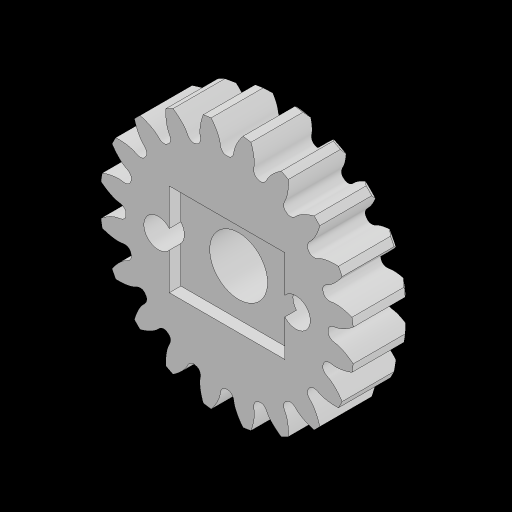
# Autodesk Inventor part: Servo Gear
Saved by Autodesk Inventor 2023.2 (Build 272271030, 271C)
## iProperties
Created: 2023-11-19
Part Number: Servo Gear
Material: Generic
Document SubType Name: Modeling
Designer: robpl
Density: 1 g/cm^3
Appearance: Default
Author: robpl
## iProperties of the stored document Servo Gear_3DPrint.ipt
Created: 2023-11-27
Part Number: Servo Gear_3DPrint
Material: Generic
Document SubType Name: Modeling
Designer: robpl
Density: 1 g/cm^3
Appearance: Default
Author: robpl
Autodesk Inventor part; units mm, degrees
ref_plane "YZ Plane" through (0, 0, 0) normal (1, 0, 0) x (0, 1, 0)
ref_plane "XZ Plane" through (0, 0, 0) normal (0, 1, 0) x (-1, 0, 0)
ref_plane "XY Plane" through (0, 0, 0) normal (0, 0, 1) x (1, 0, 0)
sketch "Sketch1" plane through (0, 0, 0) normal (0, 0, 1) x (1, 0, 0)
  spline S0 degree 3 poles (-1.3768, 10.9135) (-1.3419, 10.869) (-1.2721, 10.78) (-1.173, 10.6424) (-1.0781, 10.5017) (-0.9884, 10.3578) (-0.9041, 10.2106) (-0.826, 10.06) (-0.7548, 9.906) (-0.6919, 9.7484) (-0.6476, 9.6141) (-0.6191, 9.5046) (-0.6016, 9.4215) (-0.5932, 9.3371) (-0.5774, 9.2537) (-0.5568, 9.1714) (-0.5289, 9.0912) (-0.4924, 9.0144) (-0.4469, 8.9426) (-0.4, 8.8894) (-0.3582, 8.8513) (-0.3238, 8.8264) (-0.2881, 8.8034) (-0.2496, 8.7854) (-0.2102, 8.7696) (-0.169, 8.7594) (-0.1272, 8.7515) (-0.0706, 8.7491) (0, 8.7506) (0.0706, 8.7491) (0.1272, 8.7515) (0.169, 8.7594) (0.2102, 8.7696) (0.2496, 8.7854) (0.2881, 8.8034) (0.3238, 8.8264) (0.3582, 8.8513) (0.4, 8.8894) (0.4469, 8.9426) (0.4924, 9.0144) (0.5289, 9.0912) (0.5568, 9.1714) (0.5774, 9.2537) (0.5932, 9.3371) (0.6016, 9.4215) (0.6191, 9.5046) (0.6476, 9.6141) (0.6919, 9.7484) (0.7548, 9.906) (0.826, 10.06) (0.9041, 10.2106) (0.9884, 10.3578) (1.0781, 10.5017) (1.173, 10.6424) (1.2721, 10.78) (1.3419, 10.869) (1.3768, 10.9135) knots 0 0 0 0 0.01696 0.03392 0.050881 0.067841 0.084801 0.101761 0.11872 0.135679 0.152636 0.161116 0.169595 0.178075 0.186555 0.195032 0.203511 0.211989 0.220465 0.228938 0.233179 0.237417 0.241658 0.245897 0.250137 0.254376 0.258616 0.262855 0.271335 0.279816 0.284054 0.288295 0.292534 0.296774 0.301013 0.305254 0.309492 0.313732 0.322205 0.330682 0.33916 0.347638 0.356116 0.364596 0.373076 0.381555 0.390034 0.406992 0.423951 0.44091 0.45787 0.47483 0.49179 0.50875 0.52571 0.54267 0.54267 0.54267 0.54267
  circle A0 centre (0, 0) radius 8.75 construction
  circle A1 centre (0, 0) radius 9.3969 construction
  circle A2 centre (0, 0) radius 10 construction
  circle A3 centre (0, 0) radius 11
  point P0 (-1.2731, 10.7793)
  point P1 (-1.1737, 10.6419)
  point P2 (-1.079, 10.5012)
  point P3 (-0.9893, 10.3573)
  point P4 (-0.9051, 10.21)
  point P5 (-0.8271, 10.0594)
  point P6 (-0.7562, 9.9054)
  point P7 (-0.6935, 9.7478)
  point P8 (-0.641, 9.5865)
  point P9 (-0.6197, 9.5045)
  point P10 (-0.6031, 9.4213)
  point P11 (-0.592, 9.3373)
  point P12 (-0.5766, 9.2539)
  point P13 (-0.5556, 9.1717)
  point P14 (-0.5275, 9.0917)
  point P15 (-0.4909, 9.0153)
  point P16 (-0.4451, 8.9439)
  point P17 (-0.3892, 8.8802)
  point P18 (-0.3577, 8.8519)
  point P19 (-0.3236, 8.8267)
  point P20 (-0.2876, 8.8042)
  point P21 (-0.2495, 8.7858)
  point P22 (-0.2099, 8.7705)
  point P23 (-0.1689, 8.7598)
  point P24 (-0.1271, 8.7525)
  point P25 (-0.0848, 8.75)
  point P26 (0, 8.75)
  point P27 (0.0848, 8.75)
  point P28 (0.1271, 8.7525)
  point P29 (0.1689, 8.7598)
  point P30 (0.2099, 8.7705)
  point P31 (0.2495, 8.7858)
  point P32 (0.2876, 8.8042)
  point P33 (0.3236, 8.8267)
  point P34 (0.3577, 8.8519)
  point P35 (0.3892, 8.8802)
  point P36 (0.4451, 8.9439)
  point P37 (0.4909, 9.0153)
  point P38 (0.5275, 9.0917)
  point P39 (0.5556, 9.1717)
  point P40 (0.5766, 9.2539)
  point P41 (0.592, 9.3373)
  point P42 (0.6031, 9.4213)
  point P43 (0.6197, 9.5045)
  point P44 (0.641, 9.5865)
  point P45 (0.6935, 9.7478)
  point P46 (0.7562, 9.9054)
  point P47 (0.8271, 10.0594)
  point P48 (0.9051, 10.21)
  point P49 (0.9893, 10.3573)
  point P50 (1.079, 10.5012)
  point P51 (1.1737, 10.6419)
  point P52 (1.2731, 10.7793)
  constraints: 4 centre point, 2 point on circle, 115 other
extrude "Extrusion1" add sketch "Sketch1" against normal blind 5
extrude "Extrusion2" cut sketch "Sketch1" against normal through all contours A3 S0 picked at (-0.172, 10.4001)
pattern_circular "Circular Pattern1" count 20 over 360 about axis through (0, 0, 0) along (0, 0, -1) of "Extrusion2"
sketch "Sketch2" plane through (0, 0, -5) normal (0, 0, -1) x (-1, 0, 0)
  line L0 (-5.95, 0) -> (5.95, 0)
  point P0 (0, 0)
  point P1 (0, 0)
  dimension "d7" = 11.9
  constraints: 3 coincident, 2 end point, 1 horizontal, 1 midpoint
  measures "d7" distance of L0.start L0.end
hole "Hole1" at (5.95, 0, -5) at (-5.95, 0, -5) direction (0, 0, 1) diameter 2.5 end through all counterbore diameter 5.5 counterbore depth 2
sketch "Sketch3" plane through (0, 0, -5) normal (0, 0, -1) x (-1, 0, 0)
  point P0 (0, 0)
  point P1 (0, 0)
  constraints: 1 coincident
hole "Hole2" at (0, 0, -5) direction (0, 0, 1) diameter 5 end through all
sketch "Sketch6" plane through (0, 0, 0) normal (0, 1, 0) x (-1, 0, 0)
  line L0 (-2.5, 0) -> (2.5, 0) projected
  line L1 (2.5, -5) -> (-2.5, -5) projected
  line L2 (0, -5) -> (-11, -5)
  line L3 (-11, -5) -> (-11, -4.5)
  line L4 (-11, -4.5) -> (-10.5, -5)
  line L5 (0, -6.4043) -> (0, 3.4007) projected
  point P0 (0, 0)
  dimension "d33" = 11
  dimension "d34" = 0.5
  dimension "d35" = 0.5
  constraints: 6 end point, 1 point on line, 1 vertical
  measures "d33" distance of L2.start L2.end
  measures "d34" distance of L2.end L3.end
  measures "d35" distance of L4.end L2.end
revolve "Revolution2" cut sketch "Sketch6" angle 360 about axis through (0, 0, -10) along (0, 0, 1)
sketch "Sketch7" plane through (0, 0, 0) normal (0, 0, 1) x (1, 0, 0)
  line L0 (5, -4) -> (-5, -4)
  line L1 (-5, -4) -> (-5, 4)
  line L2 (-5, 4) -> (5, 4)
  line L3 (5, 4) -> (5, -4)
  line L4 (5, -4) -> (-5, 4) construction
  line L5 (-5, -4) -> (5, 4) construction
  point P0 (0, 0)
  dimension "d37" = 10
  dimension "d38" = 8
  constraints: 12 end point, 2 midpoint, 2 parallel, 1 horizontal, 1 perpendicular
  measures "d37" distance of L1.end L2.end
  measures "d38" distance of L0.end L1.end
extrude "Extrusion4" cut sketch "Sketch7" against normal blind 1
equation "\"d0\" = FaceWidth"
equation "\"d35\" = d34"
equation "\"Module\" = 1"
equation "\"PressureAngle\" = 20deg"
equation "\"UnitProfileClearance\" = 0.25"
equation "\"UnitRoundRadius\" = 0.35"
equation "\"HeadDiameter\" = 22"
equation "\"RootDiameter\" = 17.5"
equation "\"BaseDiameter\" = 18.79385"
equation "\"FaceWidth\" = 5"
equation "\"HelixAngle\" = 0"
equation "\"UnitCorrection\" = 0"
equation "\"UnitAddendumModification\" = 0"
equation "\"CircularPitch\" = 3.141593"
equation "\"UnitBacklashShift\" = 0"
equation "\"TotalToolShift\" = 0"
equation "\"IsInternal\" = 0"
body "Solid1"
